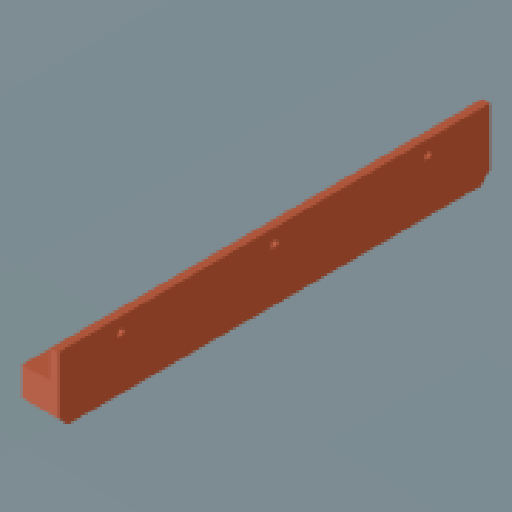
# Autodesk Inventor part: Toolhead Dock Assembly
Saved by Autodesk Inventor 2023.2 (Build 272271000, 271)
## iProperties
Created: 2023-02-06
Part Number: Toolhead Dock Assembly
Material: ABS Plastic
Document SubType Name: Modeling
Designer: remop
Density: 1.06 g/cm^3
Appearance: Smooth - Light Orange
Author: remop
Autodesk Inventor part; units mm, degrees
ref_plane "YZ Plane" through (0, 0, 0) normal (1, 0, 0) x (0, 1, 0)
ref_plane "XZ Plane" through (0, 0, 0) normal (0, 1, 0) x (-1, 0, 0)
ref_plane "XY Plane" through (0, 0, 0) normal (0, 0, 1) x (1, 0, 0)
sketch "Sketch1" plane through (0, 0, 0) normal (0, 0, 1) x (1, 0, 0)
  line L0 (0, 0) -> (0, 15)
  line L1 (0, 15) -> (4, 15)
  line L2 (4, 15) -> (4, -20)
  line L3 (4, -20) -> (-15, -20)
  line L4 (-15, -20) -> (-15, 0)
  line L5 (-15, 0) -> (0, 0)
  dimension "d0" = 15
  dimension "d1" = 4
  dimension "d2" = 35
  constraints: 12 end point, 6 perpendicular, 1 vertical
  measures "d0" distance of L0.start L0.end
  measures "d1" distance of L0.end L1.end
  measures "d2" distance of L1.end L2.end
extrude "Extrusion1" add sketch "Sketch1" along normal blind 225
sketch "Sketch2" plane through (4, -20, 0) normal (1, 0, 0) x (0, 0, -1)
  line L0 (0, 0) -> (0, 35) projected
  line L1 (0, 35) -> (-225, 35) projected
  line L2 (-225, 0) -> (-225, 35) projected
  line L3 (0, 0) -> (-225, 0) projected
  point P0 (0, 20)
  point P1 (-192.5, 27.5)
  point P2 (-112.5, 27.5)
  point P3 (-32.5, 27.5)
  point P4 (-112.5, 35)
  dimension "d5" = 80
  dimension "d6" = 80
  dimension "d7" = 7.5
  constraints: 2 horizontal alignment, 1 midpoint, 1 vertical alignment
  measures "d5" distance of point (-112.5, 27.5) point (-192.5, 27.5)
  measures "d6" distance of point (-32.5, 27.5) point (-112.5, 27.5)
  measures "d7" distance from line of L1 point (-112.5, 27.5)
hole "Hole1" at (4, 7.5, 192.5) at (4, 7.5, 112.5) at (4, 7.5, 32.5) direction (-1, 0, 0) diameter 3.5 end through all
chamfer "Chamfer1" distance 5 angle 45 2 edges at (-5.5, -20, 225) (-5.5, -20, 0)
sketch "Sketch3" plane through (-15, 0, 0) normal (-1, 0, 0) x (0, 0, 1)
  line L0 (5, -20) -> (220, -20) projected
  line L1 (225, -15) -> (220, -20) projected
  line L2 (225, 0) -> (225, -15) projected
  line L3 (5, -20) -> (0, -15) projected
  line L4 (0, 0) -> (0, -15) projected
  line L5 (0, 0) -> (225, 0) projected
  point P0 (32.5, -10)
  point P1 (112.5, -10)
  point P2 (192.5, -10)
  point P3 (112.5, -20)
  dimension "d18" = 80
  dimension "d19" = 80
  dimension "d20" = 10
  constraints: 2 horizontal alignment, 1 midpoint, 1 vertical alignment
  measures "d18" distance of point (192.5, -10) point (112.5, -10)
  measures "d19" distance of point (32.5, -10) point (112.5, -10)
  measures "d20" distance from line of L5 point (112.5, -10)
hole "Hole2" at (-15, -10, 32.5) at (-15, -10, 112.5) at (-15, -10, 192.5) direction (1, 0, 0) diameter 2.8 depth 15
equation "\"d6\" = d5"
equation "\"d19\" = d18"
body "Solid1"
